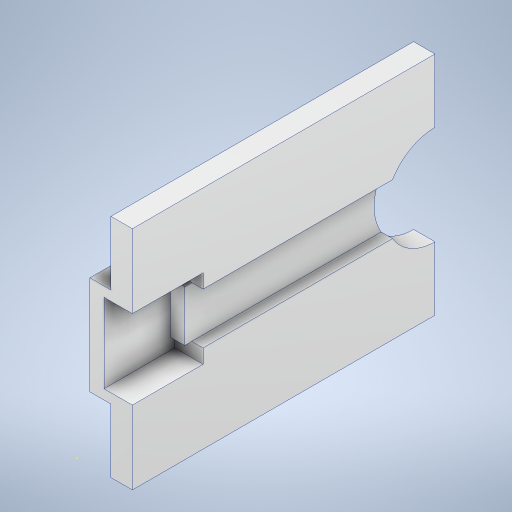
# Autodesk Inventor part: MainRails
Saved by Autodesk Inventor 2024 (Build 280153000, 153)
## iProperties
Created: 2023-08-20
Part Number: MainRails
Material: Aluminum 6061
Document SubType Name: Modeling
Designer: KirikDK
Mass: 3062.81 g
Surface Area: 1947.42 cm^2
Volume: 1134.37 cm^3
Density: 2.7 g/cm^3
Appearance: Aluminum - Flat
Author: KirikDK
Autodesk Inventor part; units mm, degrees
ref_plane "YZ Plane" through (0, 0, 0) normal (1, 0, 0) x (0, 1, 0)
ref_plane "XZ Plane" through (0, 0, 0) normal (0, 1, 0) x (-1, 0, 0)
ref_plane "XY Plane" through (0, 0, 0) normal (0, 0, 1) x (1, 0, 0)
sketch "Sketch1" plane through (0, 0, 0) normal (0, 1, 0) x (-1, 0, 0)
  line L0 (0, 279.3478) -> (-39.1304, 279.3478)
  line L1 (-39.1304, 279.3478) -> (-39.1304, -270.6522)
  line L2 (-39.1304, -270.6522) -> (0, -270.6522)
  line L3 (0, -270.6522) -> (0, 279.3478)
  line L4 (-39.1304, 279.3478) -> (-29.1304, 279.3478)
  line L5 (-29.1304, 254.3478) -> (-39.1304, 254.3478)
  line L6 (-39.1304, 254.3478) -> (-39.1304, 279.3478)
  line L7 (-39.1304, -270.6522) -> (-29.1304, -270.6522)
  line L8 (-29.1304, -245.6522) -> (-39.1304, -245.6522)
  line L9 (-39.1304, -245.6522) -> (-39.1304, -270.6522)
  point P0 (0, 0)
  point P1 (-39.1304, 254.3478)
  point P2 (-39.1304, -245.6522)
  dimension "d0" = 550
  dimension "d4" = 25
  dimension "d5" = 25
  dimension "d28" = 39.1304
  constraints: 20 end point, 4 parallel, 3 horizontal, 1 perpendicular
  measures "d0" distance of L2.end L0.start
  measures "d4" distance between parallel lines of L0 L5
  measures "d5" distance between parallel lines of L2 L8
  measures "d28" distance of L0.start L0.end
extrude "Extrusion1" add sketch "Sketch1" along normal blind 160
sketch "Sketch2" plane through (0, 0, 279.3478) normal (0, 0, 1) x (1, 0, 0)
  line L0 (0, 160) -> (39.1304, 160) projected
  line L1 (0, 160) -> (39.1304, 160)
  line L2 (39.1304, 160) -> (39.1304, 0)
  line L3 (39.1304, 0) -> (0, 0)
  line L4 (0, 0) -> (0, 160)
  line L5 (39.1304, 160) -> (39.1304, 160)
  line L6 (39.1304, 160) -> (39.1304, 115)
  line L7 (39.1304, 115) -> (39.1304, 115)
  line L8 (39.1304, 115) -> (39.1304, 160)
  line L9 (39.1304, 0) -> (39.1304, 0)
  line L10 (39.1304, 0) -> (39.1304, 45)
  line L11 (39.1304, 45) -> (39.1304, 45)
  line L12 (39.1304, 45) -> (39.1304, 0)
  circle A0 centre (39.1304, 80) radius 18
  line L13 (31.1304, 75) -> (39.1304, 75)
  line L14 (39.1304, 75) -> (39.1304, 98)
  line L15 (39.1304, 98) -> (31.1304, 98)
  line L16 (31.1304, 98) -> (31.1304, 75)
  line L17 (31.1304, 75) -> (39.1304, 75)
  line L18 (39.1304, 75) -> (39.1304, 62)
  line L19 (39.1304, 62) -> (31.1304, 62)
  line L20 (31.1304, 62) -> (31.1304, 75)
  line L21 (39.1304, 0) -> (39.1304, 160) projected
  line L22 (0, 160) -> (9.1304, 160)
  line L23 (9.1304, 160) -> (9.1304, 0)
  line L24 (9.1304, 0) -> (0, 0)
  line L25 (0, 0) -> (0, 160)
  line L26 (19.1304, 98) -> (-11, 98)
  line L27 (-11, 98) -> (-11, 62)
  line L28 (-11, 62) -> (19.1304, 62)
  line L29 (19.1304, 62) -> (19.1304, 98)
  line L30 (-8, 54) -> (24, 54)
  line L31 (24, 54) -> (24, 0)
  line L32 (24, 0) -> (-8, 0)
  line L33 (-8, 0) -> (-8, 54)
  line L34 (-8, 160) -> (24, 160)
  line L35 (24, 160) -> (24, 106)
  line L36 (24, 106) -> (-8, 106)
  line L37 (-8, 106) -> (-8, 160)
  point P0 (0, 0)
  point P1 (39.1304, 115)
  point P2 (39.1304, 160)
  point P3 (39.1304, 45)
  point P4 (39.1304, 0)
  point P5 (39.1304, 115)
  point P6 (0, 98)
  point P7 (0, 62)
  point P8 (9.1304, 98)
  point P9 (9.1304, 106)
  point P10 (9.1304, 54)
  point P11 (9.1304, 62)
  dimension "d6" = 0
  dimension "d7" = 45
  dimension "d8" = 45
  dimension "d9" = 8
  dimension "d10" = 36
  dimension "d11" = 80
  dimension "d12" = 80
  dimension "d15" = 30
  dimension "d34" = 12
  constraints: 72 end point, 18 equal length, 9 horizontal, 9 perpendicular, 8 point on line, 3 midpoint, 2 point on circle, 1 centre point, 3 other
  measures "d6" distance between parallel lines of L2 L10
  measures "d7" distance between parallel lines of L11 L3
  measures "d8" distance from line of L0 point (39.13, 115)
  measures "d9" distance between parallel lines of L2 L16
  measures "d10" diameter of A0
  measures "d11" distance from line of L3 point (39.13, 80)
  measures "d12" distance of point (39.13, 160) point (39.13, 80)
  measures "d15" distance between parallel lines of L2 L23
  measures "d34" distance between parallel lines of L20 L29
extrude "Extrusion2" cut sketch "Sketch2" against normal up to surface (550 mm away) contours L0 L23 L36 L4 | L0 L35 L36 L23 | L36 L23 L26 L4 | L26 L23 L28 L4 | L26 L29 L28 L23 | L28 L23 L30 L4 | L30 L23 L3 L4 | L2 L13 L16 A0 | A0 L16 L15 | L30 L31 L3 L23 | L2 A0 L20 L13 | L19 L20 A0
sketch "Sketch5" plane through (39.1304, 160, 279.3478) normal (1, 0, 0) x (0, 0, -1)
  line L0 (0, -62) -> (0, 0) projected
  line L1 (0, -160) -> (550, -160) projected
  line L2 (0, 0) -> (214, 0)
  line L3 (214, 0) -> (214, -160)
  line L4 (214, -160) -> (0, -160)
  line L5 (0, -160) -> (0, 0)
  circle A0 centre (214, -80) radius 35
  line L6 (214, 0) -> (550, 0)
  line L7 (550, 0) -> (550, -160)
  line L8 (550, -160) -> (214, -160)
  line L9 (214, -160) -> (214, 0)
  point P0 (279.3478, -160)
  point P1 (214, -45)
  point P2 (214, -115)
  dimension "d30" = 160
  dimension "d31" = 70
  constraints: 16 end point, 4 parallel, 2 horizontal, 2 perpendicular, 1 centre point, 1 midpoint, 1 point on line
  measures "d30" distance between parallel lines of L2 L1
  measures "d31" diameter of A0
extrude "Extrusion4" cut sketch "Sketch5" against normal blind 100 contours L6 L7 L1 L3 A0 | A0 L3 | L3 A0
sketch "Sketch6" plane through (19.1304, 62, 279.3478) normal (-1, 0, 0) x (0, 0, 1)
  line L0 (0, 52.95) -> (-60, 52.95)
  line L1 (-60, 52.95) -> (-60, -16.95)
  line L2 (-60, -16.95) -> (0, -16.95)
  line L3 (0, -16.95) -> (0, 52.95)
  line L4 (0, -62) -> (-214, -62) projected
  line L5 (-214, 98) -> (0, 98) projected
  point P0 (-279.3478, -62)
  dimension "d43" = 45.05
  dimension "d44" = 45.05
  dimension "d45" = 60
  constraints: 8 end point, 2 parallel, 1 horizontal, 1 perpendicular
  measures "d43" distance between parallel lines of L2 L4
  measures "d44" distance between parallel lines of L5 L0
  measures "d45" distance of L1.end L2.end
extrude "Extrusion5" add sketch "Sketch6" along normal mid plane 20
sketch "Sketch7" plane through (24, 0, 279.3478) normal (0, 0, 1) x (1, 0, 0)
  point P0 (-24, 0)
sketch "Sketch8" plane through (39.1304, 0, 279.3478) normal (1, 0, 0) x (0, 0, -1)
  line L0 (0, 0) -> (0, 62) projected
  line L1 (0, 52) -> (50, 52)
  line L2 (50, 52) -> (50, 108)
  line L3 (50, 108) -> (0, 108)
  line L4 (0, 108) -> (0, 52)
  line L5 (183.9833, 62) -> (0, 62) projected
  line L6 (0, 98) -> (183.9833, 98) projected
  point P0 (279.3478, 0)
  dimension "d38" = 10
  dimension "d39" = 10
  dimension "d40" = 50
  constraints: 8 end point, 2 parallel, 1 horizontal, 1 perpendicular, 1 point on line
  measures "d38" distance between parallel lines of L1 L5
  measures "d39" distance between parallel lines of L3 L6
  measures "d40" distance of L2.end L3.end
extrude "Extrusion6" cut sketch "Sketch8" against normal blind 20
sketch "Sketch9" plane through (31.1304, 80, 65.3478) normal (1, 0, 0) x (0, 0, -1)
  line L0 (-164, 18) -> (-164, -18) projected
  line L1 (-154, -18) -> (-30.0167, -18) projected
  line L2 (-164, 18) -> (-169, 18)
  line L3 (-169, 18) -> (-169, -18)
  line L4 (-169, -18) -> (-164, -18)
  line L5 (-164, -18) -> (-164, 18)
  point P0 (65.3478, -80)
  point P1 (-214, -18)
  constraints: 8 end point, 2 parallel, 1 horizontal, 1 perpendicular, 1 point on line
extrude "Extrusion7" add sketch "Sketch9" against normal blind 10
sketch "Sketch10" plane through (9.1304, 45.05, 279.3478) normal (-1, 0, 0) x (0, 0, 1)
  line L0 (-60, 52.95) -> (-60, 16.95) projected
  line L1 (-60, 26.95) -> (-65, 26.95)
  line L2 (-65, 26.95) -> (-65, 42.95)
  line L3 (-65, 42.95) -> (-60, 42.95)
  line L4 (-60, 42.95) -> (-60, 26.95)
  line L5 (-60, 16.95) -> (-183.9833, 16.95) projected
  line L6 (-60, 52.95) -> (-183.9833, 52.95) projected
  point P0 (-279.3478, -45.05)
  point P1 (-60, 42.95)
  dimension "d48" = 10
  dimension "d49" = 10
  constraints: 8 end point, 2 parallel, 1 horizontal, 1 perpendicular, 1 point on line
  measures "d48" distance between parallel lines of L5 L1
  measures "d49" distance between parallel lines of L3 L6
extrude "Extrusion8" add sketch "Sketch10" against normal blind 10
body "Solid1"
